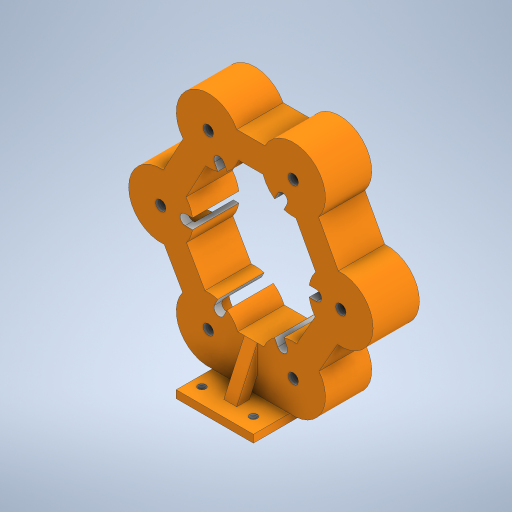
# Autodesk Inventor part: support_under beams_2022
Saved by Autodesk Inventor 2023 (Build 270158000, 158)
## iProperties
Created: 2019-08-12
Part Number: support_under beams_2022
Material: Generic
Document SubType Name: Modeling
Designer: shenglab2
Density: 1 g/cm^3
Appearance: Default
Author: shenglab2
Autodesk Inventor part; units mm, degrees
ref_plane "YZ Plane" through (0, 0, 0) normal (1, 0, 0) x (0, 1, 0)
ref_plane "XZ Plane" through (0, 0, 0) normal (0, 1, 0) x (-1, 0, 0)
ref_plane "XY Plane" through (0, 0, 0) normal (0, 0, 1) x (1, 0, 0)
sketch "Sketch1" plane through (0, 0, 0) normal (0, 0, 1) x (1, 0, 0)
  circle A0 centre (0, 0) radius 50
  circle A1 centre (-35, -22) radius 10.4
  circle A2 centre (35, -22) radius 10.4
  circle A3 centre (16.5, -54.5) radius 10.4
  circle A4 centre (16.5, 12.5) radius 10.4
  circle A5 centre (-16.5, 12.5) radius 10.4
  line L0 (31.5, -44) -> (1.5, -44)
  line L1 (1.5, -44) -> (1.5, -21)
  line L2 (1.5, -21) -> (31.5, -21)
  line L3 (31.5, -21) -> (31.5, -44)
  line L4 (31.5, -44) -> (1.5, -21) construction
  line L5 (1.5, -44) -> (31.5, -21) construction
  line L6 (50, -11.5) -> (20, -11.5)
  line L7 (20, -11.5) -> (20, 11.5)
  line L8 (20, 11.5) -> (50, 11.5)
  line L9 (50, 11.5) -> (50, -11.5)
  line L10 (50, -11.5) -> (20, 11.5) construction
  line L11 (20, -11.5) -> (50, 11.5) construction
  line L12 (-20, -11.5) -> (-50, -11.5)
  line L13 (-50, -11.5) -> (-50, 11.5)
  line L14 (-50, 11.5) -> (-20, 11.5)
  line L15 (-20, 11.5) -> (-20, -11.5)
  line L16 (-20, -11.5) -> (-50, 11.5) construction
  line L17 (-50, -11.5) -> (-20, 11.5) construction
  line L18 (31.5, 23) -> (1.5, 23)
  line L19 (1.5, 23) -> (1.5, 46)
  line L20 (1.5, 46) -> (31.5, 46)
  line L21 (31.5, 46) -> (31.5, 23)
  line L22 (31.5, 23) -> (1.5, 46) construction
  line L23 (1.5, 23) -> (31.5, 46) construction
  line L24 (-1.5, 23) -> (-31.5, 23)
  line L25 (-31.5, 23) -> (-31.5, 46)
  line L26 (-31.5, 46) -> (-1.5, 46)
  line L27 (-1.5, 46) -> (-1.5, 23)
  line L28 (-1.5, 23) -> (-31.5, 46) construction
  line L29 (-31.5, 23) -> (-1.5, 46) construction
  line L30 (-50, 0) -> (50, 0)
  line L31 (0, 50) -> (0, -50)
  line L32 (-35, 0) -> (-35, -22) construction
  line L33 (35, 0) -> (35, -22) construction
  line L34 (16.5, 34.5) -> (16.5, 12.5) construction
  line L35 (-16.5, 34.5) -> (-16.5, 12.5) construction
  circle A6 centre (-16.5, -54.5) radius 10.4
  line L36 (-1.5, -21) -> (-31.5, -21)
  line L37 (-1.5, -44) -> (-1.5, -21)
  line L38 (-31.5, -21) -> (-31.5, -44)
  line L39 (-1.5, -44) -> (-31.5, -21) construction
  line L40 (-31.5, -44) -> (-1.5, -21) construction
  line L41 (-31.5, -44) -> (-1.5, -44)
  circle A7 centre (0, 0) radius 70
  circle A8 centre (-16.5, 12.5) radius 12.5
  circle A9 centre (16.5, 12.5) radius 12.5
  circle A10 centre (35, -22) radius 12.5
  circle A11 centre (16.5, -54.5) radius 12.5
  circle A12 centre (-16.5, -54.5) radius 12.5
  circle A13 centre (-35, -22) radius 12.5
  line L42 (16.5, 12.5) -> (35, -22)
  line L43 (35, -22) -> (16.5, -54.5)
  line L44 (16.5, -54.5) -> (-16.5, -54.5)
  line L45 (-16.5, -54.5) -> (-35, -22)
  line L46 (-35, -22) -> (-16.5, 12.5)
  line L47 (-16.5, 12.5) -> (16.5, 12.5)
  line L48 (26.3205, 4.7664) -> (33.9924, -9.5407)
  line L49 (17.5076, 0.0407) -> (25.1795, -14.2664)
  line L50 (-26.3205, 4.7664) -> (-33.9924, -9.5407)
  line L51 (-17.5076, 0.0407) -> (-25.1795, -14.2664)
  line L52 (-24.9872, -29.4829) -> (-17.8222, -42.0701)
  line L53 (5.0436, -59.5) -> (-5.0436, -59.5)
  line L54 (5.0436, -49.5) -> (-5.0436, -49.5)
  line L55 (24.9872, -29.4829) -> (17.8222, -42.0701)
  line L56 (33.6778, -34.4299) -> (26.5128, -47.0171)
  line L57 (-26.5128, -47.0171) -> (-33.6778, -34.4299)
  line L58 (5.4641, 18.3702) -> (-5.4641, 18.3702)
  line L59 (4.7019, 8.3702) -> (-4.7019, 8.3702)
  point P0 (16.5, -32.5)
  point P1 (-35, 0)
  point P2 (-16.5, -32.5)
  point P3 (23.2823, -44)
  point P4 (23.7487, -44)
  point P5 (23.4913, -44.138)
  dimension "d0" = 100
  dimension "d16" = 30
  dimension "d17" = 23
  dimension "d20" = 30
  dimension "d21" = 23
  dimension "d22" = 30
  dimension "d23" = 23
  dimension "d24" = 30
  dimension "d25" = 23
  dimension "d26" = 30
  dimension "d27" = 23
  dimension "d30" = 22
  dimension "d31" = 22
  dimension "d32" = 1.5
  dimension "d33" = 100
  dimension "d35" = 22
  dimension "d36" = 1.5
  dimension "d37" = 22
  dimension "d38" = 20.8
  dimension "d39" = 20.8
  dimension "d40" = 1.5
  dimension "d41" = 4
  dimension "d42" = 4
  dimension "d43" = 6
  dimension "d45" = 22
  dimension "d46" = 140
  dimension "d83" = 20.8
  dimension "d84" = 20.8
  dimension "d85" = 20.8
  dimension "d87" = 25
  dimension "d88" = 25
  dimension "d89" = 25
  dimension "d90" = 25
  dimension "d91" = 25
  dimension "d92" = 25
  dimension "d99" = 5
  dimension "d100" = 5
  dimension "d101" = 5
  dimension "d102" = 5
  dimension "d103" = 5
  dimension "d104" = 5
  dimension "d105" = 5
  dimension "d106" = 5
  dimension "d107" = 5
  dimension "d108" = 5
  dimension "d109" = 10
  constraints: 120 end point, 27 point on circle, 20 parallel, 14 centre point, 14 midpoint, 8 coincident, 7 horizontal, 6 perpendicular, 6 symmetric about line, 3 vertical, 2 point on line, 2 tangent, 1 other
  measures "d0" diameter of A0
  measures "d16" distance of L2.start L2.end
  measures "d17" distance of L1.start L2.start
  measures "d20" distance of L8.start L8.end
  measures "d21" distance of L7.start L8.start
  measures "d22" distance of L14.start L14.end
  measures "d23" distance of L13.start L14.start
  measures "d24" distance of L20.start L20.end
  measures "d25" distance of L19.start L20.start
  measures "d26" distance of L26.start L26.end
  measures "d27" distance of L25.start L26.start
  measures "d30" distance of L32.start L32.end
  measures "d31" distance of L33.start L33.end
  measures "d32" distance between parallel lines of L19 L31
  measures "d33" distance of L31.start L31.end
  measures "d35" distance of L34.start L34.end
  measures "d36" distance between parallel lines of L31 L27
  measures "d37" distance of L35.start L35.end
  measures "d38" diameter of A5
  measures "d39" diameter of A4
  measures "d40" distance between parallel lines of L31 L1
  measures "d41" distance from line of L20 L31.start
  measures "d42" distance from line of L26 L31.start
  measures "d43" distance from line of L0 L31.end
  measures "d45" distance of A3.centre point (16.5, -32.5)
  measures "d46" diameter of A7
  measures "d83" diameter of A1
  measures "d84" diameter of A2
  measures "d85" diameter of A3
  measures "d87" diameter of A8
  measures "d88" diameter of A9
  measures "d89" diameter of A10
  measures "d90" diameter of A11
  measures "d91" diameter of A12
  measures "d92" diameter of A13
  measures "d99" distance between parallel lines of L42 L48
  measures "d100" distance between parallel lines of L42 L49
  measures "d101" distance between parallel lines of L46 L50
  measures "d102" distance between parallel lines of L46 L51
  measures "d103" distance between parallel lines of L45 L57
  measures "d104" distance between parallel lines of L45 L52
  measures "d105" distance between parallel lines of L44 L54
  measures "d106" distance between parallel lines of L44 L53
  measures "d107" distance between parallel lines of L43 L55
  measures "d108" distance between parallel lines of L43 L56
  measures "d109" distance between parallel lines of L59 L58
extrude "Extrusion7" add sketch "Sketch1" along normal blind 18 contours A9 L42 A4 L8 | L8 A4 L47 A9 L18 | A10 A0 A2 | A0 A2 L42 L6 A10 | L6 L42 A10 | L8 L7 L42 L47 A4 | A4 L42 L7 L8 | A2 A0 | A0 A2 L3 L43 L42 | L42 A2 L2 A10 L6 | L6 A10 L42 | A9 L7 A4 L42 | L18 A9 | A4 L7 L42 | A0 A10 L3 A2 | L42 L43 L3 L2 A2 | A9 L47 A4 L7 | A4 L47 L42 L7 | L3 A10 L43 A2 | A2 L43 L3 | L2 L3 L43 A2 | A2 L43 A10 L2 | A8 L47 A5 L14 L24 | A8 L15 A5 L47 | L24 A8 | L14 A5 L46 A8 | L47 L46 L15 L14 A5 | A5 L15 L46 L47 | L43 L0 A11 | A11 L0 L43 | A11 L44 A3 L43 A0 | A0 L43 L0 A11 | A11 L0 L43 A0 A3 | A12 A0 A6 L45 L41 | L14 L15 L46 A5 | L15 A8 L46 A5 | A5 L46 L15 | L43 A3 A0 | A12 L44 A6 A0 | A0 A3 L44 A11 | L41 L45 A12 | A13 L12 L46 A1 A0 | A0 A1 A13 | A13 L46 L12 | A3 L43 L44 A0 | A0 A3 | A3 L44 L43 | A6 L44 L45 A0 | A0 A6 | A12 A0 L45 A6 L44 | L45 A0 A12 L41 | L41 A12 L45 | A1 L46 L45 L38 A0 | A0 A1 | A0 A1 L38 A13 | L46 A13 L12 | L12 A13 L36 A1 L46 | A6 L45 A0 | A6 L45 L44 | A13 L45 A1 L36 | A1 L36 L38 L45 L46 | A13 L38 A1 L45 | L38 L45 A1 | A1 L45 L38 L36
extrude "Extrusion8" cut sketch "Sketch1" along normal blind 15 contours L8 L7 L42 L47 A4 | A4 L42 L7 L8 | A2 A0 | A0 A2 L3 L43 L42 | A4 L7 L42 | L42 L43 L3 L2 A2 | A4 L47 L42 L7 | A2 L43 L3 | L2 L3 L43 A2 | L47 L46 L15 L14 A5 | A5 L15 L46 L47 | L14 L15 L46 A5 | A5 L46 L15 | A3 L43 L44 A0 | A0 A3 | A3 L44 L43 | A6 L44 L45 A0 | A0 A6 | A1 L46 L45 L38 A0 | A0 A1 | A6 L45 L44 | A1 L36 L38 L45 L46 | L38 L45 A1 | A1 L45 L38 L36
extrude "Extrusion9" add sketch "Sketch1" along normal blind 18 contours L48 A10 L42 L30 | L30 L42 A9 L48 | L42 A10 L6 L49 L7 L30 | L30 L7 A9 L42 | L30 L49 A9 L7 | L7 L49 L30 | A10 L49 L6 | L58 A9 L47 L31 | L31 L47 A8 L58 | L56 L3 A10 | L47 A9 L59 L31 | L31 L59 A8 L47 | L3 L56 A0 L0 A11 L43 A10 | L56 L0 A0 | L43 A11 L55 A10 | L0 L56 A11 A0 | A0 A11 L0 | L54 A11 A0 L31 | L31 A0 A12 L54 | L51 L15 L30 | L30 L15 A8 L51 | A0 A11 L44 A12 | L50 A8 L46 L30 | L30 L46 A13 L50 | L30 L46 A8 L15 | L15 L51 L12 A13 L46 L30 | L53 A12 L44 A11 | L51 A13 L12 | A12 L45 A13 L52 | A12 A0 L41 | L41 A0 L57 L38 A13 L45 A12 | A13 L38 L57 | L57 L41 A0 A12 | L41 L57 A0
sketch "Sketch6" plane through (0, 0, 0) normal (0, 0, -1) x (-1, 0, 0)
  arc A0 (-26.5128, -47.0171) -> (-5.0436, -59.5) centre (-16.5, -54.5) ccw projected
  line L0 (5.0436, -59.5) -> (-5.0436, -59.5) projected
  arc A1 (5.0436, -59.5) -> (26.5128, -47.0171) centre (16.5, -54.5) ccw projected
  circle A2 centre (0, 0) radius 70 projected
  line L1 (-15, -70) -> (15, -70)
  line L2 (-15, -70) -> (-15, -66.9097)
  line L3 (15, -70) -> (15, -66.9097)
  point P0 (0, -70)
  dimension "d112" = 30
  constraints: 6 end point, 2 horizontal, 2 point on circle, 1 midpoint, 1 parallel, 1 vertical, 1 vertical alignment, 1 other
  measures "d112" distance of L1.start L1.end
extrude "Extrusion10" add sketch "Sketch6" against normal blind 18 contours A0 L0 A1 L3 A2 L2 | A2 L1 L2 | A2 L3 L1 picked at (0, -63)
sketch "Sketch7" plane through (-15, -70, 0) normal (0, -1, 0) x (1, 0, 0)
  line L0 (30, 0) -> (0, 0) projected
  line L1 (0, 0) -> (30, 18) construction
  line L2 (30, 32) -> (0, 32)
  line L3 (0, 32) -> (0, 0)
  line L4 (0, 0) -> (30, 0)
  line L5 (30, 0) -> (30, 32)
  line L6 (30, 32) -> (0, 0) construction
  line L7 (0, 32) -> (30, 0) construction
  point P0 (15, 0)
  point P1 (15, 0)
  dimension "d115" = 30
  dimension "d116" = 32
  constraints: 14 end point, 2 midpoint, 2 parallel, 1 horizontal, 1 perpendicular
  measures "d115" distance of L4.end L3.end
  measures "d116" distance of L2.end L3.end
extrude "Extrusion11" add sketch "Sketch7" against normal blind 3
sketch "Sketch9" plane through (0, 0, 18) normal (0, 0, 1) x (1, 0, 0)
  arc A0 (-17.5076, 0.0407) -> (-4.7019, 8.3702) centre (-16.5, 12.5) ccw projected
  arc A1 (4.7019, 8.3702) -> (17.5076, 0.0407) centre (16.5, 12.5) ccw projected
  arc A2 (25.1795, -14.2664) -> (24.9872, -29.4829) centre (35, -22) ccw projected
  arc A3 (17.8222, -42.0701) -> (5.0436, -49.5) centre (16.5, -54.5) ccw projected
  arc A4 (-5.0436, -49.5) -> (-17.8222, -42.0701) centre (-16.5, -54.5) ccw projected
  arc A5 (-24.9872, -29.4829) -> (-25.1795, -14.2664) centre (-35, -22) ccw projected
  arc A6 (17.8222, -42.0701) -> (5.0436, -49.5) centre (16.5, -54.5) ccw projected
  circle A7 centre (-16.5, 12.5) radius 2
  circle A8 centre (16.5, 12.5) radius 2
  circle A9 centre (-35, -22) radius 2
  circle A10 centre (35, -22) radius 2
  circle A11 centre (16.5, -54.5) radius 2
  circle A12 centre (-16.5, -54.5) radius 2
  circle A13 centre (-16.5, 12.5) radius 10.4 projected
  circle A14 centre (16.5, 12.5) radius 10.4 projected
  circle A15 centre (35, -22) radius 10.4 projected
  circle A16 centre (16.5, -54.5) radius 10.4 projected
  circle A17 centre (-16.5, -54.5) radius 10.4 projected
  circle A18 centre (-35, -22) radius 10.4 projected
  line L0 (-16.5, 12.5) -> (16.5, -54.5) construction
  line L1 (16.5, 12.5) -> (-16.5, -54.5) construction
  line L2 (-35, -22) -> (35, -22) construction
  line L3 (-10.9769, 1.2864) -> (-12.3024, 3.9777) construction
  line L4 (-9.1827, 2.1701) -> (-10.5082, 4.8614)
  line L5 (-14.0966, 3.094) -> (-12.7711, 0.4027)
  arc A19 (-12.7711, 0.4027) -> (-9.1827, 2.1701) centre (-10.9769, 1.2864) ccw
  arc A20 (-10.5082, 4.8614) -> (-14.0966, 3.094) centre (-12.3024, 3.9777) ccw
  line L6 (10.9769, 1.2864) -> (12.3024, 3.9777) construction
  line L7 (12.7711, 0.4027) -> (14.0966, 3.094)
  line L8 (10.5082, 4.8614) -> (9.1827, 2.1701)
  arc A21 (9.1827, 2.1701) -> (12.7711, 0.4027) centre (10.9769, 1.2864) ccw
  arc A22 (14.0966, 3.094) -> (10.5082, 4.8614) centre (12.3024, 3.9777) ccw
  arc A23 (-24.9872, -29.4829) -> (-25.1795, -14.2664) centre (-35, -22) ccw projected
  line L9 (-22.5, -22) -> (-25.5, -22) construction
  line L10 (-22.5, -20) -> (-25.5, -20)
  line L11 (-25.5, -24) -> (-22.5, -24)
  arc A24 (-22.5, -24) -> (-22.5, -20) centre (-22.5, -22) ccw
  arc A25 (-25.5, -20) -> (-25.5, -24) centre (-25.5, -22) ccw
  arc A26 (25.1795, -14.2664) -> (24.9872, -29.4829) centre (35, -22) ccw projected
  line L12 (22.5, -22) -> (25.5, -22) construction
  line L13 (22.5, -24) -> (25.5, -24)
  line L14 (25.5, -20) -> (22.5, -20)
  arc A27 (22.5, -20) -> (22.5, -24) centre (22.5, -22) ccw
  arc A28 (25.5, -24) -> (25.5, -20) centre (25.5, -22) ccw
  arc A29 (-5.0436, -49.5) -> (-17.8222, -42.0701) centre (-16.5, -54.5) ccw projected
  line L15 (-10.9769, -43.2864) -> (-12.3024, -45.9777) construction
  line L16 (-12.7711, -42.4027) -> (-14.0966, -45.094)
  line L17 (-10.5082, -46.8614) -> (-9.1827, -44.1701)
  arc A30 (-9.1827, -44.1701) -> (-12.7711, -42.4027) centre (-10.9769, -43.2864) ccw
  arc A31 (-14.0966, -45.094) -> (-10.5082, -46.8614) centre (-12.3024, -45.9777) ccw
  arc A32 (17.8222, -42.0701) -> (5.0436, -49.5) centre (16.5, -54.5) ccw projected
  line L18 (10.9769, -43.2864) -> (12.3024, -45.9777) construction
  line L19 (9.1827, -44.1701) -> (10.5082, -46.8614)
  line L20 (14.0966, -45.094) -> (12.7711, -42.4027)
  arc A33 (12.7711, -42.4027) -> (9.1827, -44.1701) centre (10.9769, -43.2864) ccw
  arc A34 (10.5082, -46.8614) -> (14.0966, -45.094) centre (12.3024, -45.9777) ccw
  point P0 (23.4913, -44.138)
  point P1 (23.2823, -44)
  point P2 (-11.6397, 2.632)
  point P3 (11.6397, 2.632)
  point P4 (-24, -22)
  point P5 (24, -22)
  point P6 (-11.6397, -44.632)
  point P7 (11.6397, -44.632)
  point P8 (-9.2539, -44.3146)
  point P9 (-12.8422, -42.5472)
  point P10 (12.8422, -42.5472)
  point P11 (9.2539, -44.3146)
  point P12 (22.661, -20)
  point P13 (22.661, -24)
  point P14 (9.2539, 2.3146)
  point P15 (12.8422, 0.5472)
  point P16 (-22.661, -24)
  point P17 (-22.661, -20)
  point P18 (-12.8422, 0.5472)
  point P19 (-9.2539, 2.3146)
  dimension "d128" = 4
  dimension "d129" = 4
  dimension "d130" = 4
  dimension "d131" = 4
  dimension "d132" = 4
  dimension "d133" = 4
  dimension "d134" = 3
  dimension "d135" = 4
  dimension "d136" = 3
  dimension "d137" = 4
  dimension "d138" = 3
  dimension "d139" = 4
  dimension "d140" = 3
  dimension "d141" = 4
  dimension "d142" = 3
  dimension "d143" = 4
  dimension "d144" = 3
  dimension "d145" = 4
  constraints: 54 end point, 30 point on circle, 24 tangent, 18 centre point, 12 point on line, 6 coincident, 6 midpoint, 6 parallel, 1 horizontal
  measures "d128" diameter of A7
  measures "d129" diameter of A8
  measures "d130" diameter of A9
  measures "d131" diameter of A10
  measures "d132" diameter of A11
  measures "d133" diameter of A12
  measures "d134" distance of L3.start L3.end
  measures "d135" diameter of A20
  measures "d136" distance of L6.start L6.end
  measures "d137" diameter of A22
  measures "d138" distance of L9.start L9.end
  measures "d139" diameter of A25
  measures "d140" distance of L12.start L12.end
  measures "d141" diameter of A28
  measures "d142" distance of L15.start L15.end
  measures "d143" diameter of A31
  measures "d144" distance of L18.start L18.end
  measures "d145" diameter of A34
extrude "Extrusion12" cut sketch "Sketch9" against normal blind 18 contours L5 A13 L4 A0 | L5 A20 L4 A13 | L8 A14 L7 A1 | L8 A22 L7 A14 | L14 A15 L13 A2 | L14 A28 L13 A15 | L20 A16 L19 A3 | L20 A34 L19 A16 | L17 A17 L16 A4 | L17 A31 L16 A17 | L11 A18 L10 A5 | L11 A25 L10 A18 | A7 | A8 | A9 | A10 | A11 | A12 picked at (-12.4082, 4.0106) picked at (12.4082, 4.0106) picked at (25.5762, -21.9196) picked at (12.4082, -46.0106) picked at (-12.4082, -46.0106) picked at (-25.4559, -22.6022)
sketch "Sketch10" plane through (0, 0, 0) normal (1, 0, 0) x (0, 1, 0)
  line L0 (-49.5, 18) -> (-67, 18) construction
  line L1 (-67, 18) -> (-67, 26) construction
  line L2 (-49.5, 18) -> (-67, 26)
  point P0 (0, 0)
  dimension "d148" = 8
  dimension "d149" = 17.5
  constraints: 6 end point, 1 horizontal, 1 perpendicular
  measures "d148" distance of L0.end L1.end
  measures "d149" distance of L0.start L0.end
extrude "Rib1" add sketch "Sketch10" along normal mid plane 5 rib yes fills toward (-58.2708, 21.9545) open curves L2
thread "Thread1" size "M4x0.7" class "6H" standard "ANSI Metric M Profile" full length
thread "Thread2" size "M4x0.7" class "6H" standard "ANSI Metric M Profile" full length
thread "Thread3" size "M4x0.7" class "6H" standard "ANSI Metric M Profile" full length
thread "Thread4" size "M4x0.7" class "6H" standard "ANSI Metric M Profile" full length
thread "Thread5" size "M4x0.7" class "6H" standard "ANSI Metric M Profile" full length
thread "Thread6" size "M4x0.7" class "6H" standard "ANSI Metric M Profile" full length
sketch "Sketch12" plane through (2.5, -67, 18) normal (1, 0, 0) x (0, 0, -1)
  line L0 (0, 0) -> (-8, 0) projected
  line L1 (0, 17.5) -> (0, 0) projected
  line L2 (-8, 0) -> (0, 17.5) projected
  line L3 (0, 6.6764) -> (-3.0521, 0)
  point P0 (18, 67)
  dimension "d176" = 4.5
  constraints: 2 end point, 2 point on line, 1 parallel
  measures "d176" distance between parallel lines of L2 L3
extrude "Extrusion14" cut sketch "Sketch12" against normal blind 10 contours L0 L3 L1
sketch "Sketch13" plane through (-15, -70, 0) normal (0, -1, 0) x (1, 0, 0)
  line L0 (30, 32) -> (30, 18) projected
  line L1 (30, 32) -> (-2, 0)
  line L2 (4, 6) -> (24, 6)
  line L3 (24, 6) -> (24, 26)
  line L4 (24, 26) -> (4, 26)
  line L5 (4, 26) -> (4, 6)
  line L6 (4, 6) -> (24, 26) construction
  line L7 (24, 6) -> (4, 26) construction
  point P0 (15, 0)
  point P1 (14, 16)
  dimension "d179" = 20
  dimension "d180" = 20
  constraints: 14 end point, 3 midpoint, 2 parallel, 1 horizontal, 1 perpendicular, 1 point on line
  measures "d179" distance of L2.end L3.end
  measures "d180" distance of L3.end L4.end
hole "Hole3" at (9, -70, 26) direction (0, 1, 0) diameter 3 end through all
hole "Hole4" at (-11, -70, 26) direction (0, 1, 0) diameter 3 end through all
thread "Thread9" size "M3x0.5" class "6H" standard "ANSI Metric M Profile" full length
thread "Thread10" size "M3x0.5" class "6H" standard "ANSI Metric M Profile" full length
body "Solid3"
